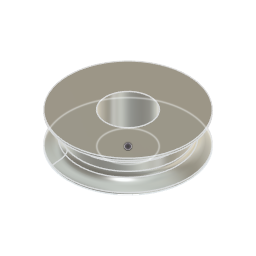
MotorHead_60AIM40F_HGR (Autodesk Fusion 360 archive; units mm, degrees)
design "Pulley_HGR"
Autodesk Fusion 360 part; units mm, degrees
note: some values were not read from the file. Set by a fixed rule: the direction of a hole.
sketch "Sketch1" plane through (0, 0, 0) normal (0, 0, 1) x (1, 0, 0)
  circle A0 centre (0, 0) radius 15
  circle A1 centre (0, 0) radius 5.55
  dimension "d1" = 30
  dimension "d6" = 11.1
  constraint coincident A0.centre A1.centre
  measures "d1" diameter of A0
  measures "d6" diameter of A1
extrude "Extrude1" add sketch "Sketch1" along normal blind 8 contours A0 | A1
ref_plane "WorkPlane1" through (-4.8884, -14.1811, 8) normal (0.945406, -0.325896, 0) x (0.325896, 0.945406, 0)
sketch "Sketch2" plane through (-4.8884, -14.1811, 8) normal (0.945406, -0.325896, 0) x (0.325896, 0.945406, 0)
  line L0 (0, -0.5) -> (0, -7.5)
  spline S0 degree 5 poles (0, -0.5) (0.0405, -0.5236) (0.1216, -0.5701) (0.2437, -0.6379) (0.4071, -0.7243) (0.6124, -0.8257) (0.8187, -0.921) (1.0259, -1.0118) (1.2333, -1.1005) (1.4403, -1.1916) (1.6462, -1.29) (1.8499, -1.4008) (2.0508, -1.5289) (2.2483, -1.6776) (2.442, -1.8483) (2.632, -2.0415) (2.781, -2.214) (2.8912, -2.3532) (2.9638, -2.4503) (3, -2.5) knots 0 0 0 0 0 0 0.066667 0.133333 0.2 0.266667 0.333333 0.4 0.466667 0.533333 0.6 0.666667 0.733333 0.8 0.866667 0.933333 1 1 1 1 1 1
  spline S1 degree 5 poles (0, -7.5) (0.0405, -7.4764) (0.1216, -7.4299) (0.2437, -7.3621) (0.4071, -7.2757) (0.6124, -7.1743) (0.8187, -7.079) (1.0259, -6.9882) (1.2333, -6.8995) (1.4403, -6.8084) (1.6462, -6.71) (1.8499, -6.5992) (2.0508, -6.4711) (2.2483, -6.3224) (2.442, -6.1517) (2.632, -5.9585) (2.781, -5.786) (2.8912, -5.6468) (2.9638, -5.5497) (3, -5.5) knots 0 0 0 0 0 0 0.066667 0.133333 0.2 0.266667 0.333333 0.4 0.466667 0.533333 0.6 0.666667 0.733333 0.8 0.866667 0.933333 1 1 1 1 1 1
  line L1 (3, -2.5) -> (3, -5.5)
  point P0 (1, -1)
  point P1 (2, -1.5)
  point P2 (1, -7)
  point P3 (2, -6.5)
  constraint vertical L0
  constraint vertical L1
revolve "Revolve1" cut sketch "Sketch2" angle 360 about axis through (0, 0, 1.75) along (0, 0, 1)
hole "Hole1" at (0, 0, 0) direction (0, 0, 1) diameter 11.2 depth 8 tip angle 118
fillet "Fillet1" radius 1.5 2 edges at (-11.1879, -4.3394, 5.5) (-11.1879, -4.3394, 2.5)

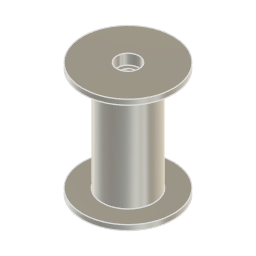
design "BushingPulley60AIM_HGR"
Autodesk Fusion 360 part; units mm, degrees
sketch "Sketch1" plane through (0, 0, 0) normal (0, 0, 1) x (1, 0, 0)
  circle A0 centre (0, 0) radius 10.05
  line L0 (2.35, -4.25) -> (2.35, -9.45)
  line L1 (-2.35, -4.25) -> (2.35, -4.25)
  line L2 (-2.35, -4.25) -> (2.35, -9.45) construction
  line L3 (2.35, -9.45) -> (-2.35, -9.45)
  line L4 (2.35, -4.25) -> (-2.35, -9.45) construction
  line L5 (-2.35, -9.45) -> (-2.35, -4.25)
  circle A1 centre (0, 0) radius 7.15
  circle A2 centre (0, 0) radius 17.5
  line L6 (0, 0) -> (0, -12)
  point P0 (0, -6.85)
  dimension "d1" = 20.1
  dimension "d2" = 4.7
  dimension "d3" = 5.2
  dimension "d4" = 14.3
  dimension "d5" = 2.9
  dimension "d10" = 35
  constraint coincident A0.centre A1.centre
  constraint horizontal L1
  constraint perpendicular L0 L1
  constraint parallel L1 L3
  constraint parallel L0 L5
  constraint coincident P0 L2
  constraint coincident P0 L4
  constraint perpendicular L3 L6
  constraint coincident P0 L6
  measures "d1" diameter of A0
  measures "d2" distance of L3.end L0.end
  measures "d3" distance of L0.end L0.start
  measures "d4" diameter of A1
  measures "d5" distance of L1 A1
  measures "d10" diameter of A2
extrude "Extrude1" add sketch "Sketch1" along normal blind 42 contours A0 | L0 L1 A1 L6 | L0 L3 A1 L6 | L1 L5 A1 L6 | L3 L5 A1 L6 makes body 1
extrude "Extrude2" add sketch "Sketch1" along normal blind 2 contours A2 bodies 1
extrude "Extrude3" add sketch "Sketch1" along normal blind 2 from surface at 42 separate body contours A0 | L0 L1 A1 L6 | L0 L3 A1 L6 | L1 L5 A1 L6 | L3 L5 A1 L6 | A2 makes body 2
extrude "Extrude4" add sketch "Sketch1" against normal blind 20 from surface at 44 separate body contours L0 L1 L5 A1 | L0 L1 A1 L6 | L1 L5 A1 L6 makes body 3
combine "Combine1" operation add target body 2 tool bodies 3
move_face "OffsetFaces1" [suppressed]
sketch "Sketch2" plane through (0, 0, 44) normal (0, 0, 1) x (-1, 0, 0)
  circle A0 centre (0, 0) radius 17.5
  circle A1 centre (0, 0) radius 3
  constraint concentric A0 A1
extrude "Extrude5" cut sketch "Sketch1" against normal blind 18 from surface at 42 contours L0 L1 A1 L6 | L1 L5 A1 L6 bodies 1
hole "Hole1" at (0, 0, 44) direction (0, 0, -1) diameter 5.4 depth 65 tip angle 118 counterbore diameter 8.6 counterbore depth 4 bodies 2
extrude "Extrude6" cut sketch "Sketch1" along normal blind 7 contours L0 L1 A1 L6 | L1 L5 A1 L6 bodies 1

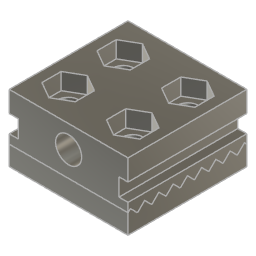
design "60AIMTensioner"
Autodesk Fusion 360 part; units mm, degrees
sketch "Sketch1" plane through (0, 0, 0) normal (1, 0, 0) x (0, 1, 0)
  line L0 (-15, 0) -> (-13.5, 1.5)
  line L1 (-13.5, 1.5) -> (-12, 0)
  line L2 (-12, 0) -> (-10.5, 1.5)
  line L3 (-10.5, 1.5) -> (-9, 0)
  line L4 (-9, 0) -> (-7.5, 1.5)
  line L5 (-7.5, 1.5) -> (-6, 0)
  line L6 (-6, 0) -> (-4.5, 1.5)
  line L7 (-4.5, 1.5) -> (-3, 0)
  line L8 (-3, 0) -> (-1.5, 1.5)
  line L9 (-1.5, 1.5) -> (0, 0)
  line L10 (0, 0) -> (1.5, 1.5)
  line L11 (1.5, 1.5) -> (3, 0)
  line L12 (3, 0) -> (4.5, 1.5)
  line L13 (4.5, 1.5) -> (6, 0)
  line L14 (6, 0) -> (7.5, 1.5)
  line L15 (7.5, 1.5) -> (9, 0)
  line L16 (9, 0) -> (10.5, 1.5)
  line L17 (10.5, 1.5) -> (12, 0)
  line L18 (11, 0) -> (11, -3.1)
  line L19 (11, -3.1) -> (-14, -3.1)
  line L20 (-14, -3.1) -> (-14, 0)
  line L21 (-14, 0) -> (-14, 1)
  line L22 (11, 0) -> (11, 1)
  line L23 (11, 0) -> (11, 11)
  line L24 (11, 11) -> (-14, 11)
  line L25 (-14, 11) -> (-14, 0)
  dimension "d4" = 24
  dimension "d5" = 0
  dimension "d6" = 3.1
  dimension "d7" = 11
  constraint perpendicular L0 L1
  constraint vertical L18
  constraint horizontal L19
  constraint vertical L20
  constraint coincident L0 L21.end
  constraint coincident L17 L22.end
  constraint vertical L23
  constraint horizontal L24
  constraint vertical L25
  measures "d6" distance of L20.end L19.end
  measures "d7" distance of L20.end L24.end
extrude "Extrude1" add sketch "Sketch1" along normal blind 25 contours L0 L1 L2 L3 L4 L5 L6 L7 L8 L9 L10 L11 L12 L13 L14 L15 L16 L17 L18 L19 L20 L21 L22 L23 L25 makes body 1
extrude "Extrude2" add sketch "Sketch1" along normal blind 25 separate body contours L0 L1 L2 L3 L4 L5 L6 L7 L8 L9 L10 L11 L12 L13 L14 L15 L16 L17 L23 L24 L25 makes body 2
sketch "Sketch2" plane through (0, 11, 0) normal (0, 1, 0) x (-1, 0, 0)
  line L0 (0, 1) -> (0, 11)
  line L1 (0, 11) -> (-25, 11)
  line L2 (-25, 11) -> (-25, 1)
  line L3 (-25, 1) -> (0, 1)
  circle A0 centre (-12.5, 6.25) radius 2.75
  line L4 (-7.8813, 6.2268) -> (-10.1705, 10.2383)
  line L5 (-10.1705, 10.2383) -> (-14.7893, 10.2616)
  line L6 (-14.7893, 10.2616) -> (-17.1187, 6.2732)
  line L7 (-17.1187, 6.2732) -> (-14.8295, 2.2617)
  line L8 (-14.8295, 2.2617) -> (-10.2107, 2.2384)
  line L9 (-10.2107, 2.2384) -> (-7.8813, 6.2268)
  point P0 (-12.5, 6.25)
  point P1 (-12.5, 6.25)
  point P2 (-12.5, 6.25)
  dimension "d12" = 5.5
  dimension "d15" = 2.5
  dimension "d16" = 12.5
  dimension "d18" = 4
  constraint coincident P2 P1
  measures "d12" diameter of A0
  measures "d15" distance of L3 A0
  measures "d16" distance of L0 P2
  measures "d18" distance of P2 L9
hole "Hole1" at (12.5, 11, 6.25) direction (0, -1, 0) diameter 5.5 depth 36.5 tip angle 118 bodies 2
extrude "Extrude3" cut sketch "Sketch2" against normal blind 4 contours L4 L5 L6 L7 L8 L9 bodies 2
sketch "Sketch3" plane through (25, 0, 0) normal (1, 0, 0) x (0, 1, 0)
  line L0 (-14, 11) -> (-14, 1)
  line L1 (-14, 1) -> (-13.5, 1.5)
  line L2 (-13.5, 1.5) -> (-12, 0)
  line L3 (-12, 0) -> (-10.5, 1.5)
  line L4 (-10.5, 1.5) -> (-9, 0)
  line L5 (-9, 0) -> (-7.5, 1.5)
  line L6 (-7.5, 1.5) -> (-6, 0)
  line L7 (-6, 0) -> (-4.5, 1.5)
  line L8 (-4.5, 1.5) -> (-3, 0)
  line L9 (-3, 0) -> (-1.5, 1.5)
  line L10 (-1.5, 1.5) -> (0, 0)
  line L11 (0, 0) -> (1.5, 1.5)
  line L12 (1.5, 1.5) -> (3, 0)
  line L13 (3, 0) -> (4.5, 1.5)
  line L14 (4.5, 1.5) -> (6, 0)
  line L15 (6, 0) -> (7.5, 1.5)
  line L16 (7.5, 1.5) -> (9, 0)
  line L17 (9, 0) -> (10.5, 1.5)
  line L18 (10.5, 1.5) -> (11, 1)
  line L19 (11, 1) -> (11, 11)
  line L20 (11, 11) -> (-14, 11)
  line L21 (-14, 3) -> (11, 3)
  line L22 (11, 3) -> (11, 6.5)
  line L23 (11, 6.5) -> (-14, 6.5)
  line L24 (-14, 6.5) -> (-14, 3)
  dimension "d28" = 25
  dimension "d29" = 3.5
  dimension "d35" = 1.5
  constraint horizontal L21
  constraint vertical L22
  constraint horizontal L23
  constraint vertical L24
  constraint coincident L0 L21.start
  measures "d28" distance of L21.start L21.end
  measures "d29" distance of L21.start L23.end
  measures "d35" distance of L1.end L21
extrude "Extrude4" cut sketch "Sketch3" against normal blind 1.9 contours L0 L19 L21 L22 L23 L24 bodies 2
extrude "Extrude5" cut sketch "Sketch3" along normal blind 1.9 from surface at -25 contours L0 L19 L21 L22 L23 L24 bodies 2
sketch "Sketch4" plane through (0, 0, -3.1) normal (0, 0, -1) x (1, 0, 0)
  line L0 (0, 14) -> (0, -11)
  line L1 (0, -11) -> (25, -11)
  line L2 (25, -11) -> (25, 14)
  line L3 (25, 14) -> (0, 14)
  circle A0 centre (19.3, -4.3) radius 2.2
  line L4 (19.3, -8.3415) -> (22.8, -6.3207)
  line L5 (22.8, -6.3207) -> (22.8, -2.2793)
  line L6 (22.8, -2.2793) -> (19.3, -0.2585)
  line L7 (19.3, -0.2585) -> (15.8, -2.2793)
  line L8 (15.8, -2.2793) -> (15.8, -6.3207)
  line L9 (15.8, -6.3207) -> (19.3, -8.3415)
  line L10 (2.2, 9.3207) -> (2.2, 5.2793)
  circle A1 centre (5.7, 7.3) radius 2.2
  line L11 (9.2, 5.2793) -> (9.2, 9.3207)
  line L12 (9.2, 9.3207) -> (5.7, 11.3415)
  line L13 (2.2, 5.2793) -> (5.7, 3.2585)
  line L14 (5.7, 3.2585) -> (9.2, 5.2793)
  line L15 (5.7, 11.3415) -> (2.2, 9.3207)
  line L16 (2.2, -2.2793) -> (2.2, -6.3207)
  line L17 (2.2, -6.3207) -> (5.7, -8.3415)
  line L18 (9.2, -2.2793) -> (5.7, -0.2585)
  line L19 (5.7, -0.2585) -> (2.2, -2.2793)
  line L20 (9.2, -6.3207) -> (9.2, -2.2793)
  circle A2 centre (5.7, -4.3) radius 2.2
  line L21 (5.7, -8.3415) -> (9.2, -6.3207)
  line L22 (12.5, 14) -> (12.5, -11)
  line L23 (0, 1.5) -> (25, 1.5)
  line L24 (15.8, 9.3207) -> (15.8, 5.2793)
  circle A3 centre (19.3, 7.3) radius 2.2
  line L25 (22.8, 5.2793) -> (22.8, 9.3207)
  line L26 (22.8, 9.3207) -> (19.3, 11.3415)
  line L27 (15.8, 5.2793) -> (19.3, 3.2585)
  line L28 (19.3, 3.2585) -> (22.8, 5.2793)
  line L29 (19.3, 11.3415) -> (15.8, 9.3207)
  point P0 (19.3, -4.3)
  point P1 (19.3, -4.3)
  point P2 (19, -4.2)
  point P3 (19, -4.2)
  point P4 (6, 7.8)
  point P5 (6, 7.8)
  point P6 (5.7, 7.3)
  point P7 (5.7, 7.3)
  point P8 (5.7, -4.3)
  point P9 (5.7, -4.3)
  point P10 (6, -4.2)
  point P11 (6, -4.2)
  point P12 (19, 8.8)
  point P13 (19, 8.8)
  point P14 (19.3, 7.3)
  point P15 (19.3, 7.3)
  dimension "d36" = 4.4
  dimension "d38" = 4.5
  dimension "d49" = 3.5
  dimension "d52" = 2.2
  dimension "d61" = 4.4
  dimension "d62" = 3.5
  dimension "d63" = 4.4
  dimension "d64" = 3.5
  dimension "d69" = 4.4
  dimension "d70" = 3.5
  constraint coincident P1 P0
  constraint parallel L2 L5
  constraint coincident P7 P6
  constraint coincident P9 P8
  constraint midpoint L3 L22.start
  constraint midpoint L1 L22.end
  constraint midpoint L0 L23.start
  constraint midpoint L2 L23.end
  constraint coincident P15 P14
  constraint symmetric P1 L23 P15
  constraint symmetric P1 P9 L22
  constraint symmetric P7 L22 P15
  constraint parallel L0 L10
  constraint parallel L0 L16
  constraint parallel L2 L25
  measures "d36" diameter of A0
  measures "d38" distance of L1 A0
  measures "d49" distance of P1 L9
  measures "d52" distance of L2 L5
  measures "d61" diameter of A1
  measures "d62" distance of P7 L13
  measures "d63" diameter of A2
  measures "d64" distance of P9 L17
  measures "d69" diameter of A3
  measures "d70" distance of P15 L27
hole "Hole2" at (19.3, 4.3, -3.1) at (5.7, 4.3, -3.1) at (19.3, -7.3, -3.1) at (5.7, -7.3, -3.1) direction (0, 0, 1) diameter 4.4 depth 36.5 tip angle 118 counterbore diameter 7.8 counterbore depth 2.5 bodies 1 2
extrude "Extrude6" cut sketch "Sketch4" along normal blind 3.5 from surface at -14.1 contours A0 | L4 L5 L6 L7 L8 L9 | L10 L11 L12 L13 L14 L15 | L16 L17 L18 L19 L20 L21 | L24 L25 L26 L27 L28 L29 bodies 2
move_face "OffsetFaces1" offset -0.1 4 faces at (0.6333, 2.6667, 3) (0.6333, -5.6667, 6.5) (23.7333, 2.6667, 3) (23.7333, -5.6667, 6.5) on bodies 2
